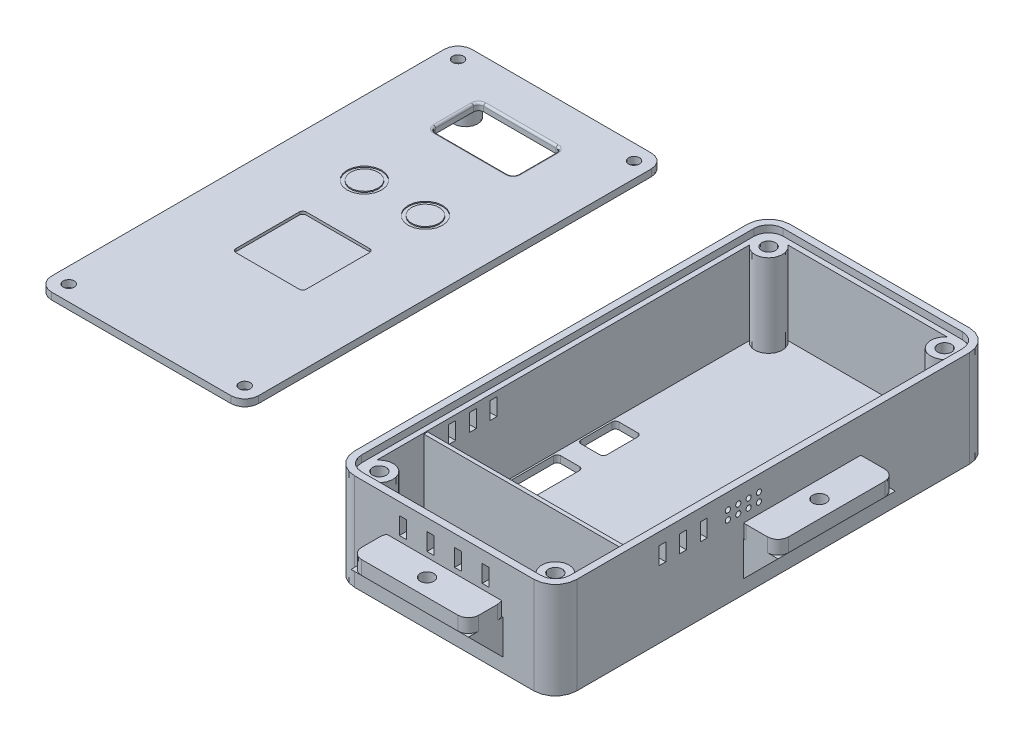
CARA_TEO (Autodesk Fusion 360 design; units mm, degrees)
part number: 2026-09-04-16-03-50-091
Autodesk Fusion 360 part; units mm, degrees
sketch "Boceto21" plane through (0, 0, 0) normal (0, 0, 1) x (1, 0, 0)
  line L0 (4, -16.8) -> (56, -16.8)
  line L1 (60, -12.8) -> (60, 101)
  line L2 (56, 105) -> (4, 105)
  line L3 (0, 101) -> (0, -12.8)
  arc A0 (56, -16.8) -> (60, -12.8) centre (56, -12.8) ccw
  arc A1 (60, 101) -> (56, 105) centre (56, 101) ccw
  arc A2 (4, 105) -> (0, 101) centre (4, 101) ccw
  arc A3 (0, -12.8) -> (4, -16.8) centre (4, -12.8) ccw
  constraint coincident L1.start A0.end
  constraint coincident L3.end A3.start
extrude "Extruir20" add sketch "Boceto21" along normal blind 2 makes body 1
sketch "Boceto22" plane through (0, 0, 0) normal (0, 0, 1) x (1, 0, 0)
  circle A0 centre (48.4706, 8.7122) radius 3.5
  circle A1 centre (11.3516, 8.7122) radius 3.5
  circle A2 centre (48.5136, 96.0852) radius 3.5
  circle A3 centre (11.0776, 96.1372) radius 3.5
extrude "Extruir21" add sketch "Boceto22" against normal blind 7 bodies 1
sketch "Boceto23" plane through (0, 0, 0) normal (0, 0, 1) x (1, 0, 0)
  circle A0 centre (48.4706, 8.7122) radius 1.25
  circle A1 centre (11.3516, 8.7122) radius 1.25
  circle A2 centre (48.5136, 96.0852) radius 1.25
  circle A3 centre (11.0776, 96.1372) radius 1.25
extrude "Extruir22" cut sketch "Boceto23" against normal blind 7 bodies 1
sketch "Boceto24" plane through (0, 0, 0) normal (0, 0, 1) x (1, 0, 0)
  circle A0 centre (4.5, -12.3) radius 1.6
  circle A1 centre (55.5, -12.3) radius 1.6
  circle A2 centre (4.5, 100.5) radius 1.6
  circle A3 centre (55.5, 100.5) radius 1.6
extrude "Extruir23" cut sketch "Boceto24" along normal blind 2 bodies 1
sketch "Boceto25" plane through (0, 0, 0) normal (0, 0, 1) x (1, 0, 0)
  line L0 (17.9336, 79.0164) -> (41.9336, 79.0164)
  line L1 (41.9336, 79.0164) -> (41.9336, 93.0164)
  line L2 (41.9336, 93.0164) -> (17.9336, 93.0164)
  line L3 (17.9336, 93.0164) -> (17.9336, 79.0164)
extrude "Extruir24" cut sketch "Boceto25" along normal blind 2 bodies 1
sketch "Boceto26" plane through (0, 0, 0) normal (0, 0, 1) x (1, 0, 0)
  line L0 (14.7446, 48.1164) -> (27.7446, 48.1164)
  line L1 (27.7446, 48.1164) -> (27.7446, 65.1164)
  line L2 (27.7446, 65.1164) -> (14.7446, 65.1164)
  line L3 (14.7446, 65.1164) -> (14.7446, 48.1164)
  line L4 (32.4246, 48.1164) -> (45.4246, 48.1164)
  line L5 (45.4246, 48.1164) -> (45.4246, 65.1164)
  line L6 (45.4246, 65.1164) -> (32.4246, 65.1164)
  line L7 (32.4246, 65.1164) -> (32.4246, 48.1164)
extrude "Extruir25" cut sketch "Boceto26" along normal blind 1.1 bodies 1
sketch "Boceto27" plane through (0, 0, 0) normal (0, 0, 1) x (1, 0, 0)
  line L0 (8.4354, 5.9164) -> (114.4697, 5.9164)
  line L1 (114.4697, 5.9164) -> (114.4697, 99.0836)
  line L2 (114.4697, 99.0836) -> (8.4354, 99.0836)
  line L3 (8.4354, 99.0836) -> (8.4354, 5.9164)
ref_plane "PlanoDeObra2" through (0, 0, 2) normal (0, 0, 1) x (1, 0, 0)
sketch "Boceto28" plane through (0, 0, 2) normal (0, 0, 1) x (1, 0, 0)
  line L0 (20.8, 19.8) -> (39.2, 19.8)
  line L1 (40.2, 20.8) -> (40.2, 39.2)
  line L2 (39.2, 40.2) -> (20.8, 40.2)
  line L3 (19.8, 39.2) -> (19.8, 20.8)
  arc A0 (39.2, 19.8) -> (40.2, 20.8) centre (39.2, 20.8) ccw
  arc A1 (40.2, 39.2) -> (39.2, 40.2) centre (39.2, 39.2) ccw
  arc A2 (20.8, 40.2) -> (19.8, 39.2) centre (20.8, 39.2) ccw
  arc A3 (19.8, 20.8) -> (20.8, 19.8) centre (20.8, 20.8) ccw
extrude "Extruir26" cut sketch "Boceto28" against normal blind 0.8 bodies 1
sketch "Boceto29" plane through (0, 0, 2) normal (0, 0, 1) x (1, 0, 0)
  circle A0 centre (21.2446, 56.6164) radius 5
  circle A1 centre (21.2446, 56.6164) radius 4
  line L0 (19.7446, 56.6164) -> (22.7446, 56.6164)
  line L1 (21.2446, 55.1164) -> (21.2446, 58.1164)
  circle A2 centre (38.9246, 56.6164) radius 5
  circle A3 centre (38.9246, 56.6164) radius 4
  line L2 (37.4246, 56.6164) -> (40.4246, 56.6164)
  line L3 (38.9246, 55.1164) -> (38.9246, 58.1164)
sketch "Boceto30" plane through (0, 0, 2) normal (0, 0, 1) x (1, 0, 0)
  circle A0 centre (21.2446, 56.6164) radius 5
  circle A1 centre (21.2446, 56.6164) radius 4
  circle A2 centre (38.9246, 56.6164) radius 5
  circle A3 centre (38.9246, 56.6164) radius 4
extrude "Extruir27" cut sketch "Boceto30" against normal blind 0.3 bodies 1
sketch "Boceto31" plane through (0, 0, 0) normal (0, 0, 1) x (1, 0, 0)
  line L0 (94, -19) -> (146, -19)
  line L1 (152.2, -12.8) -> (152.2, 101)
  line L2 (146, 107.2) -> (94, 107.2)
  line L3 (87.8, 101) -> (87.8, -12.8)
  arc A0 (146, -19) -> (152.2, -12.8) centre (146, -12.8) ccw
  arc A1 (152.2, 101) -> (146, 107.2) centre (146, 101) ccw
  arc A2 (94, 107.2) -> (87.8, 101) centre (94, 101) ccw
  arc A3 (87.8, -12.8) -> (94, -19) centre (94, -12.8) ccw
  constraint tangent L0 A0
  constraint tangent L1 A0
  constraint tangent L1 A1
  constraint tangent L2 A1
  constraint tangent L2 A2
  constraint tangent L3 A2
  constraint tangent L3 A3
  constraint tangent L0 A3
extrude "C_Cuerpo_macizo" add sketch "Boceto31" along normal blind 2 and the other way blind 26 separate body makes body 2
sketch "Boceto32" plane through (0, 0, 0) normal (0, 0, 1) x (1, 0, 0)
  line L0 (94, -17) -> (146, -17)
  line L1 (150.2, -12.8) -> (150.2, 101)
  line L2 (146, 105.2) -> (94, 105.2)
  line L3 (89.8, 101) -> (89.8, -12.8)
  arc A0 (146, -17) -> (150.2, -12.8) centre (146, -12.8) ccw
  arc A1 (150.2, 101) -> (146, 105.2) centre (146, 101) ccw
  arc A2 (94, 105.2) -> (89.8, 101) centre (94, 101) ccw
  arc A3 (89.8, -12.8) -> (94, -17) centre (94, -12.8) ccw
  constraint tangent L0 A0
  constraint tangent L1 A0
  constraint tangent L1 A1
  constraint tangent L2 A1
  constraint tangent L2 A2
  constraint tangent L3 A2
  constraint tangent L3 A3
  constraint tangent L0 A3
extrude "C_Rebaje_cara" cut sketch "Boceto32" along normal blind 2 bodies 2
sketch "Boceto33" plane through (0, 0, 0) normal (0, 0, 1) x (1, 0, 0)
  line L0 (94, -17) -> (146, -17)
  line L1 (148.7, -14.3) -> (148.7, 101)
  line L2 (146, 103.7) -> (94, 103.7)
  line L3 (91.3, 101) -> (91.3, -14.3)
  arc A0 (146, -17) -> (148.7, -14.3) centre (146, -14.3) ccw
  arc A1 (148.7, 101) -> (146, 103.7) centre (146, 101) ccw
  arc A2 (94, 103.7) -> (91.3, 101) centre (94, 101) ccw
  arc A3 (91.3, -14.3) -> (94, -17) centre (94, -14.3) ccw
  constraint tangent L0 A0
  constraint tangent L1 A0
  constraint tangent L1 A1
  constraint tangent L2 A1
  constraint tangent L2 A2
  constraint tangent L3 A2
  constraint tangent L3 A3
  constraint tangent L0 A3
extrude "C_Cavidad" cut sketch "Boceto33" against normal blind 24 bodies 2
sketch "Boceto34" plane through (0, 0, 0) normal (0, 0, 1) x (1, 0, 0)
  circle A0 centre (94.5, -12.3) radius 4
  circle A1 centre (145.5, -12.3) radius 4
  circle A2 centre (94.5, 100.5) radius 4
  circle A3 centre (145.5, 100.5) radius 4
extrude "C_Torres_esquina" add sketch "Boceto34" against normal blind 24 bodies 2
sketch "Boceto35" plane through (0, 0, 0) normal (0, 0, 1) x (1, 0, 0)
  circle A0 centre (94.5, -12.3) radius 2
  circle A1 centre (145.5, -12.3) radius 2
  circle A2 centre (94.5, 100.5) radius 2
  circle A3 centre (145.5, 100.5) radius 2
extrude "C_Pilotos_M3" cut sketch "Boceto35" against normal blind 10 bodies 2
move_body "C_Montaje_en_cara" bodies 2 to x (1, 0, 0) y (0, 1, 0) z (0, 0, 1) at (-90, 0, 0)
sketch "Boceto36" plane through (0, 0, 0) normal (1, 0, 0) x (0, 0, -1)
  line L0 (19.5, 15.9) -> (7.5, 15.9)
  line L1 (7.5, 15.9) -> (7.5, 41.9)
  line L2 (7.5, 41.9) -> (19.5, 41.9)
  line L3 (19.5, 41.9) -> (19.5, 15.9)
extrude "C_Hueco_borneras" [suppressed]
sketch "Boceto37" plane through (0, 0, 0) normal (1, 0, 0) x (0, 0, -1)
  line L0 (19.5, 43) -> (7.5, 43)
  line L1 (7.5, 43) -> (7.5, 59)
  line L2 (7.5, 59) -> (19.5, 59)
  line L3 (19.5, 59) -> (19.5, 43)
extrude "C_Hueco_USBC" [suppressed]
sketch "Boceto38" plane through (0, 0, 0) normal (1, 0, 0) x (0, 0, -1)
  line L0 (19.5, 16.55) -> (7.5, 16.55)
  line L1 (7.5, 16.55) -> (7.5, 26.85)
  line L2 (7.5, 26.85) -> (19.5, 26.85)
  line L3 (19.5, 26.85) -> (19.5, 16.55)
extrude "C_Hueco_alimentacion" [suppressed]
move_body "C_Separar_piezas" bodies 2 to x (1, 0, 0) y (0, 1, 0) z (0, 0, 1) at (90, 0, 0)
sketch "Boceto39" plane through (0, 0, 0) normal (1, 0, 0) x (0, 0, -1)
  line L0 (19.5, 47.8) -> (7.5, 47.8)
  line L1 (7.5, 47.8) -> (7.5, 58.8)
  line L2 (7.5, 58.8) -> (19.5, 58.8)
  line L3 (19.5, 58.8) -> (19.5, 47.8)
extrude "C_Hueco_sensor" [suppressed]
sketch "Boceto40" plane through (0, 0, 0) normal (0, 0, 1) x (1, 0, 0)
  line L0 (106, -29) -> (134, -29)
  line L1 (137, -26) -> (137, -20.5)
  line L2 (134, -17.5) -> (106, -17.5)
  line L3 (103, -20.5) -> (103, -26)
  arc A0 (134, -29) -> (137, -26) centre (134, -26) ccw
  arc A1 (137, -20.5) -> (134, -17.5) centre (134, -20.5) ccw
  arc A2 (106, -17.5) -> (103, -20.5) centre (106, -20.5) ccw
  arc A3 (103, -26) -> (106, -29) centre (106, -26) ccw
  line L4 (106, 105) -> (134, 105)
  line L5 (137, 108) -> (137, 114.2)
  line L6 (134, 117.2) -> (106, 117.2)
  line L7 (103, 114.2) -> (103, 108)
  arc A4 (134, 105) -> (137, 108) centre (134, 108) ccw
  arc A5 (137, 114.2) -> (134, 117.2) centre (134, 114.2) ccw
  arc A6 (106, 117.2) -> (103, 114.2) centre (106, 114.2) ccw
  arc A7 (103, 108) -> (106, 105) centre (106, 108) ccw
  constraint tangent L0 A0
  constraint tangent L1 A0
  constraint tangent L1 A1
  constraint tangent L2 A1
  constraint tangent L2 A2
  constraint tangent L3 A2
  constraint tangent L3 A3
  constraint tangent L0 A3
  constraint tangent L4 A4
  constraint tangent L5 A4
  constraint tangent L5 A5
  constraint tangent L6 A5
  constraint tangent L6 A6
  constraint tangent L7 A6
  constraint tangent L7 A7
  constraint tangent L4 A7
extrude "C_Orejas_correa" add sketch "Boceto40" along normal blind 4 from surface at -12 bodies 2
sketch "Boceto41" plane through (0, 0, 0) normal (0, 0, 1) x (1, 0, 0)
  line L0 (108.5, -9.2) -> (131.5, -9.2)
  line L1 (133, -7.7) -> (133, -6.7)
  line L2 (131.5, -5.2) -> (108.5, -5.2)
  line L3 (107, -6.7) -> (107, -7.7)
  arc A0 (131.5, -9.2) -> (133, -7.7) centre (131.5, -7.7) ccw
  arc A1 (133, -6.7) -> (131.5, -5.2) centre (131.5, -6.7) ccw
  arc A2 (108.5, -5.2) -> (107, -6.7) centre (108.5, -6.7) ccw
  arc A3 (107, -7.7) -> (108.5, -9.2) centre (108.5, -7.7) ccw
  line L4 (108.5, 110.2) -> (131.5, 110.2)
  line L5 (133, 111.7) -> (133, 112.7)
  line L6 (131.5, 114.2) -> (108.5, 114.2)
  line L7 (107, 112.7) -> (107, 111.7)
  arc A4 (131.5, 110.2) -> (133, 111.7) centre (131.5, 111.7) ccw
  arc A5 (133, 112.7) -> (131.5, 114.2) centre (131.5, 112.7) ccw
  arc A6 (108.5, 114.2) -> (107, 112.7) centre (108.5, 112.7) ccw
  arc A7 (107, 111.7) -> (108.5, 110.2) centre (108.5, 111.7) ccw
  constraint tangent L0 A0
  constraint tangent L1 A0
  constraint tangent L1 A1
  constraint tangent L2 A1
  constraint tangent L2 A2
  constraint tangent L3 A2
  constraint tangent L3 A3
  constraint tangent L0 A3
  constraint tangent L4 A4
  constraint tangent L5 A4
  constraint tangent L5 A5
  constraint tangent L6 A5
  constraint tangent L6 A6
  constraint tangent L7 A6
  constraint tangent L7 A7
  constraint tangent L4 A7
extrude "C_Ranuras_correa" [suppressed]
delete_face "SuprimirCaras1" [suppressed]
sketch "Boceto42" plane through (0, 0, 0) normal (0, 0, 1) x (1, 0, 0)
  line L0 (80.8, 35.5) -> (87, 35.5)
  line L1 (90, 38.5) -> (90, 66.5)
  line L2 (87, 69.5) -> (80.8, 69.5)
  line L3 (77.8, 66.5) -> (77.8, 38.5)
  arc A0 (87, 35.5) -> (90, 38.5) centre (87, 38.5) ccw
  arc A1 (90, 66.5) -> (87, 69.5) centre (87, 66.5) ccw
  arc A2 (80.8, 69.5) -> (77.8, 66.5) centre (80.8, 66.5) ccw
  arc A3 (77.8, 38.5) -> (80.8, 35.5) centre (80.8, 38.5) ccw
  line L4 (153, 35.5) -> (159.2, 35.5)
  line L5 (162.2, 38.5) -> (162.2, 66.5)
  line L6 (159.2, 69.5) -> (153, 69.5)
  line L7 (150, 66.5) -> (150, 38.5)
  arc A4 (159.2, 35.5) -> (162.2, 38.5) centre (159.2, 38.5) ccw
  arc A5 (162.2, 66.5) -> (159.2, 69.5) centre (159.2, 66.5) ccw
  arc A6 (153, 69.5) -> (150, 66.5) centre (153, 66.5) ccw
  arc A7 (150, 38.5) -> (153, 35.5) centre (153, 38.5) ccw
  constraint tangent L0 A0
  constraint tangent L1 A0
  constraint tangent L1 A1
  constraint tangent L2 A1
  constraint tangent L2 A2
  constraint tangent L3 A2
  constraint tangent L3 A3
  constraint tangent L0 A3
  constraint tangent L4 A4
  constraint tangent L5 A4
  constraint tangent L5 A5
  constraint tangent L6 A5
  constraint tangent L6 A6
  constraint tangent L7 A6
  constraint tangent L7 A7
  constraint tangent L4 A7
extrude "C_Orejas_laterales" add sketch "Boceto42" along normal blind 4 from surface at -12 bodies 2
sketch "Boceto43" plane through (0, 0, 0) normal (0, 0, 1) x (1, 0, 0)
  line L0 (82.3, 39.5) -> (83.3, 39.5)
  line L1 (84.8, 41) -> (84.8, 64)
  line L2 (83.3, 65.5) -> (82.3, 65.5)
  line L3 (80.8, 64) -> (80.8, 41)
  arc A0 (83.3, 39.5) -> (84.8, 41) centre (83.3, 41) ccw
  arc A1 (84.8, 64) -> (83.3, 65.5) centre (83.3, 64) ccw
  arc A2 (82.3, 65.5) -> (80.8, 64) centre (82.3, 64) ccw
  arc A3 (80.8, 41) -> (82.3, 39.5) centre (82.3, 41) ccw
  line L4 (156.7, 39.5) -> (157.7, 39.5)
  line L5 (159.2, 41) -> (159.2, 64)
  line L6 (157.7, 65.5) -> (156.7, 65.5)
  line L7 (155.2, 64) -> (155.2, 41)
  arc A4 (157.7, 39.5) -> (159.2, 41) centre (157.7, 41) ccw
  arc A5 (159.2, 64) -> (157.7, 65.5) centre (157.7, 64) ccw
  arc A6 (156.7, 65.5) -> (155.2, 64) centre (156.7, 64) ccw
  arc A7 (155.2, 41) -> (156.7, 39.5) centre (156.7, 41) ccw
  constraint tangent L0 A0
  constraint tangent L1 A0
  constraint tangent L1 A1
  constraint tangent L2 A1
  constraint tangent L2 A2
  constraint tangent L3 A2
  constraint tangent L3 A3
  constraint tangent L0 A3
  constraint tangent L4 A4
  constraint tangent L5 A4
  constraint tangent L5 A5
  constraint tangent L6 A5
  constraint tangent L6 A6
  constraint tangent L7 A6
  constraint tangent L7 A7
  constraint tangent L4 A7
extrude "C_Ranuras_laterales" [suppressed]
sketch "Boceto44" plane through (0, 0, 0) normal (0, 0, 1) x (1, 0, 0)
  line L0 (94, -0.2) -> (146, -0.2)
  line L1 (150.2, 4) -> (150.2, 101)
  line L2 (146, 105.2) -> (94, 105.2)
  line L3 (89.8, 101) -> (89.8, 4)
  arc A0 (146, -0.2) -> (150.2, 4) centre (146, 4) ccw
  arc A1 (150.2, 101) -> (146, 105.2) centre (146, 101) ccw
  arc A2 (94, 105.2) -> (89.8, 101) centre (94, 101) ccw
  arc A3 (89.8, 4) -> (94, -0.2) centre (94, 4) ccw
  constraint tangent L0 A0
  constraint tangent L1 A0
  constraint tangent L1 A1
  constraint tangent L2 A1
  constraint tangent L2 A2
  constraint tangent L3 A2
  constraint tangent L3 A3
  constraint tangent L0 A3
extrude "C_Rebaje_limpieza" [suppressed]
move_body "C_Montaje_final" bodies 2 to x (1, 0, 0) y (0, 1, 0) z (0, 0, 1) at (-90, 0, 0)
move_body "C_Separar_vista" bodies 2 to x (1, 0, 0) y (0, 1, 0) z (0, 0, 1) at (90, 0, 0)
sketch "Boceto45" plane through (0, 0, 0) normal (0, 0, 1) x (1, 0, 0)
  line L0 (92.8, 15.9) -> (98.3, 15.9)
  line L1 (99.3, 16.9) -> (99.3, 40.9)
  line L2 (98.3, 41.9) -> (92.8, 41.9)
  line L3 (91.8, 40.9) -> (91.8, 16.9)
  arc A0 (98.3, 15.9) -> (99.3, 16.9) centre (98.3, 16.9) ccw
  arc A1 (99.3, 40.9) -> (98.3, 41.9) centre (98.3, 40.9) ccw
  arc A2 (92.8, 41.9) -> (91.8, 40.9) centre (92.8, 40.9) ccw
  arc A3 (91.8, 16.9) -> (92.8, 15.9) centre (92.8, 16.9) ccw
  line L4 (92.8, 47.8) -> (98.3, 47.8)
  line L5 (99.3, 48.8) -> (99.3, 57.8)
  line L6 (98.3, 58.8) -> (92.8, 58.8)
  line L7 (91.8, 57.8) -> (91.8, 48.8)
  arc A4 (98.3, 47.8) -> (99.3, 48.8) centre (98.3, 48.8) ccw
  arc A5 (99.3, 57.8) -> (98.3, 58.8) centre (98.3, 57.8) ccw
  arc A6 (92.8, 58.8) -> (91.8, 57.8) centre (92.8, 57.8) ccw
  arc A7 (91.8, 48.8) -> (92.8, 47.8) centre (92.8, 48.8) ccw
  line L8 (141.7, 15.9) -> (147.2, 15.9)
  line L9 (148.2, 16.9) -> (148.2, 40.9)
  line L10 (147.2, 41.9) -> (141.7, 41.9)
  line L11 (140.7, 40.9) -> (140.7, 16.9)
  arc A8 (147.2, 15.9) -> (148.2, 16.9) centre (147.2, 16.9) ccw
  arc A9 (148.2, 40.9) -> (147.2, 41.9) centre (147.2, 40.9) ccw
  arc A10 (141.7, 41.9) -> (140.7, 40.9) centre (141.7, 40.9) ccw
  arc A11 (140.7, 16.9) -> (141.7, 15.9) centre (141.7, 16.9) ccw
  line L12 (141.7, 47.8) -> (147.2, 47.8)
  line L13 (148.2, 48.8) -> (148.2, 57.8)
  line L14 (147.2, 58.8) -> (141.7, 58.8)
  line L15 (140.7, 57.8) -> (140.7, 48.8)
  arc A12 (147.2, 47.8) -> (148.2, 48.8) centre (147.2, 48.8) ccw
  arc A13 (148.2, 57.8) -> (147.2, 58.8) centre (147.2, 57.8) ccw
  arc A14 (141.7, 58.8) -> (140.7, 57.8) centre (141.7, 57.8) ccw
  arc A15 (140.7, 48.8) -> (141.7, 47.8) centre (141.7, 48.8) ccw
  constraint tangent L0 A0
  constraint tangent L1 A0
  constraint tangent L1 A1
  constraint tangent L2 A1
  constraint tangent L2 A2
  constraint tangent L3 A2
  constraint tangent L3 A3
  constraint tangent L0 A3
  constraint tangent L4 A4
  constraint tangent L5 A4
  constraint tangent L5 A5
  constraint tangent L6 A5
  constraint tangent L6 A6
  constraint tangent L7 A6
  constraint tangent L7 A7
  constraint tangent L4 A7
  constraint tangent L8 A8
  constraint tangent L9 A8
  constraint tangent L9 A9
  constraint tangent L10 A9
  constraint tangent L10 A10
  constraint tangent L11 A10
  constraint tangent L11 A11
  constraint tangent L8 A11
  constraint tangent L12 A12
  constraint tangent L13 A12
  constraint tangent L13 A13
  constraint tangent L14 A13
  constraint tangent L14 A14
  constraint tangent L15 A14
  constraint tangent L15 A15
  constraint tangent L12 A15
extrude "C_Salidas_fondo" cut sketch "Boceto45" along normal blind 4 from surface at -27 bodies 2
sketch "Boceto46" plane through (0, 0, 0) normal (0, 0, 1) x (1, 0, 0)
  circle A0 centre (120, -24) radius 2
  circle A1 centre (120, 112.2) radius 2
  circle A2 centre (82.8, 52.5) radius 2
  circle A3 centre (157.2, 52.5) radius 2
extrude "C_Huecos_tornillo_orejas" cut sketch "Boceto46" along normal blind 6 from surface at -13 bodies 2
fillet "Redondeo_esquinas_OLED" radius 1.5 4 edges at (41.9336, 93.0164, 1) (17.9336, 93.0164, 1) (41.9336, 79.0164, 1) (17.9336, 79.0164, 1) on bodies 1
fillet "Suavizado_borde_OLED" radius 0.6 64 edges at (18.3729, 79.4557, 2) (29.9336, 79.0164, 2) (41.4943, 79.4557, 2) (41.9336, 86.0164, 2) (41.4943, 92.5771, 2) (29.9336, 93.0164, 2) (18.3729, 92.5771, 2) (17.9336, 86.0164, 2) (17.9336, 86.0164, 2) (18.3729, 92.5771, 2) (29.9336, 93.0164, 2) (41.4943, 92.5771, 2) (41.9336, 86.0164, 2) (41.4943, 79.4557, 2) (29.9336, 79.0164, 2) (18.3729, 79.4557, 2) (41.4943, 79.4557, 2) (41.9336, 86.0164, 2) (41.4943, 92.5771, 2) (29.9336, 93.0164, 2) (18.3729, 92.5771, 2) (17.9336, 86.0164, 2) (18.3729, 79.4557, 2) (29.9336, 79.0164, 2) (29.9336, 79.0164, 2) (18.3729, 79.4557, 2) (17.9336, 86.0164, 2) (18.3729, 92.5771, 2) (29.9336, 93.0164, 2) (41.4943, 92.5771, 2) (41.9336, 86.0164, 2) (41.4943, 79.4557, 2) (18.3729, 92.5771, 2) (17.9336, 86.0164, 2) (18.3729, 79.4557, 2) (29.9336, 79.0164, 2) (41.4943, 79.4557, 2) (41.9336, 86.0164, 2) (41.4943, 92.5771, 2) (29.9336, 93.0164, 2) (29.9336, 93.0164, 2) (41.4943, 92.5771, 2) (41.9336, 86.0164, 2) (41.4943, 79.4557, 2) (29.9336, 79.0164, 2) (18.3729, 79.4557, 2) (17.9336, 86.0164, 2) (18.3729, 92.5771, 2) (41.4943, 92.5771, 2) (29.9336, 93.0164, 2) (18.3729, 92.5771, 2) (17.9336, 86.0164, 2) (18.3729, 79.4557, 2) (29.9336, 79.0164, 2) (41.4943, 79.4557, 2) (41.9336, 86.0164, 2) (41.9336, 86.0164, 2) (41.4943, 79.4557, 2) (29.9336, 79.0164, 2) (18.3729, 79.4557, 2) (17.9336, 86.0164, 2) (18.3729, 92.5771, 2) (29.9336, 93.0164, 2) (41.4943, 92.5771, 2) on bodies 1
sketch "Boceto47" plane through (0, 0, 0) normal (0, 0, 1) x (1, 0, 0)
  line L0 (90.8, -14.3) -> (94.5, -14.3)
  line L1 (94.5, -14.3) -> (94.5, -10.3)
  line L2 (94.5, -10.3) -> (90.8, -10.3)
  line L3 (90.8, -10.3) -> (90.8, -14.3)
  line L4 (145.5, -14.3) -> (149.2, -14.3)
  line L5 (149.2, -14.3) -> (149.2, -10.3)
  line L6 (149.2, -10.3) -> (145.5, -10.3)
  line L7 (145.5, -10.3) -> (145.5, -14.3)
  line L8 (90.8, 98.5) -> (94.5, 98.5)
  line L9 (94.5, 98.5) -> (94.5, 102.5)
  line L10 (94.5, 102.5) -> (90.8, 102.5)
  line L11 (90.8, 102.5) -> (90.8, 98.5)
  line L12 (145.5, 98.5) -> (149.2, 98.5)
  line L13 (149.2, 98.5) -> (149.2, 102.5)
  line L14 (149.2, 102.5) -> (145.5, 102.5)
  line L15 (145.5, 102.5) -> (145.5, 98.5)
  line L16 (92.5, 100.5) -> (96.5, 100.5)
  line L17 (96.5, 100.5) -> (96.5, 104.2)
  line L18 (96.5, 104.2) -> (92.5, 104.2)
  line L19 (92.5, 104.2) -> (92.5, 100.5)
  line L20 (143.5, 100.5) -> (147.5, 100.5)
  line L21 (147.5, 100.5) -> (147.5, 104.2)
  line L22 (147.5, 104.2) -> (143.5, 104.2)
  line L23 (143.5, 104.2) -> (143.5, 100.5)
extrude "C_Union_torres_pared" add sketch "Boceto47" against normal blind 24 bodies 2
sketch "Boceto48" plane through (0, 0, 0) normal (0, 0, 1) x (1, 0, 0)
  circle A0 centre (94.5, -12.3) radius 2
  circle A1 centre (145.5, -12.3) radius 2
  circle A2 centre (94.5, 100.5) radius 2
  circle A3 centre (145.5, 100.5) radius 2
extrude "C_Pilotos_repaso" cut sketch "Boceto48" against normal blind 10 bodies 2
sketch "Boceto49" plane through (0, 0, 0) normal (0, 0, 1) x (1, 0, 0)
  line L0 (92.5, -17.5) -> (96.5, -17.5)
  line L1 (96.5, -17.5) -> (96.5, -12.3)
  line L2 (96.5, -12.3) -> (92.5, -12.3)
  line L3 (92.5, -12.3) -> (92.5, -17.5)
  line L4 (143.5, -17.5) -> (147.5, -17.5)
  line L5 (147.5, -17.5) -> (147.5, -12.3)
  line L6 (147.5, -12.3) -> (143.5, -12.3)
  line L7 (143.5, -12.3) -> (143.5, -17.5)
extrude "C_Union_torres_extremo" add sketch "Boceto49" against normal blind 24 bodies 2
sketch "Boceto50" plane through (0, 0, 0) normal (0, 0, 1) x (1, 0, 0)
  circle A0 centre (94.5, -12.3) radius 2
  circle A1 centre (145.5, -12.3) radius 2
extrude "C_Pilotos_repaso_extremo" cut sketch "Boceto50" against normal blind 10 bodies 2
sketch "Boceto51" plane through (0, 0, 0) normal (1, 0, 0) x (0, 0, -1)
  circle A0 centre (2.5, 31) radius 0.75
  circle A1 centre (5, 31) radius 0.75
  circle A2 centre (2.5, 34) radius 0.75
  circle A3 centre (5, 34) radius 0.75
  circle A4 centre (2.5, 37) radius 0.75
  circle A5 centre (5, 37) radius 0.75
  circle A6 centre (2.5, 40) radius 0.75
  circle A7 centre (5, 40) radius 0.75
extrude "C_Agujeros_buzzer" cut sketch "Boceto51" along normal blind 10 from surface at 146 bodies 2
sketch "Boceto52" plane through (0, 0, 0) normal (1, 0, 0) x (0, 0, -1)
  line L0 (6.5, 11) -> (1.5, 11)
  line L1 (1.5, 11) -> (1.5, 13)
  line L2 (1.5, 13) -> (6.5, 13)
  line L3 (6.5, 13) -> (6.5, 11)
  line L4 (6.5, 17) -> (1.5, 17)
  line L5 (1.5, 17) -> (1.5, 19)
  line L6 (1.5, 19) -> (6.5, 19)
  line L7 (6.5, 19) -> (6.5, 17)
  line L8 (6.5, 23) -> (1.5, 23)
  line L9 (1.5, 23) -> (1.5, 25)
  line L10 (1.5, 25) -> (6.5, 25)
  line L11 (6.5, 25) -> (6.5, 23)
extrude "C_Ventilacion_lat_Xmenos" cut sketch "Boceto52" along normal blind 10 from surface at 84 bodies 2
sketch "Boceto53" plane through (0, 0, 0) normal (1, 0, 0) x (0, 0, -1)
  line L0 (6.5, 11) -> (1.5, 11)
  line L1 (1.5, 11) -> (1.5, 13)
  line L2 (1.5, 13) -> (6.5, 13)
  line L3 (6.5, 13) -> (6.5, 11)
  line L4 (6.5, 17) -> (1.5, 17)
  line L5 (1.5, 17) -> (1.5, 19)
  line L6 (1.5, 19) -> (6.5, 19)
  line L7 (6.5, 19) -> (6.5, 17)
  line L8 (6.5, 23) -> (1.5, 23)
  line L9 (1.5, 23) -> (1.5, 25)
  line L10 (1.5, 25) -> (6.5, 25)
  line L11 (6.5, 25) -> (6.5, 23)
extrude "C_Ventilacion_lat_Xmas" cut sketch "Boceto53" along normal blind 10 from surface at 146 bodies 2
ref_plane "PlanoDeObra3" through (0, -18, 0) normal (0, 1, 0) x (0, 0, 1)
sketch "Boceto54" plane through (0, -18, 0) normal (0, 1, 0) x (1, 0, 0)
  line L0 (107, 6.5) -> (109, 6.5)
  line L1 (109, 6.5) -> (109, 1.5)
  line L2 (109, 1.5) -> (107, 1.5)
  line L3 (107, 1.5) -> (107, 6.5)
  line L4 (115, 6.5) -> (117, 6.5)
  line L5 (117, 6.5) -> (117, 1.5)
  line L6 (117, 1.5) -> (115, 1.5)
  line L7 (115, 1.5) -> (115, 6.5)
  line L8 (123, 6.5) -> (125, 6.5)
  line L9 (125, 6.5) -> (125, 1.5)
  line L10 (125, 1.5) -> (123, 1.5)
  line L11 (123, 1.5) -> (123, 6.5)
  line L12 (131, 6.5) -> (133, 6.5)
  line L13 (133, 6.5) -> (133, 1.5)
  line L14 (133, 1.5) -> (131, 1.5)
  line L15 (131, 1.5) -> (131, 6.5)
extrude "C_Ventilacion_convertidor" cut sketch "Boceto54" along normal mid plane 6 bodies 2
sketch "Boceto55" plane through (0, 0, 0) normal (1, 0, 0) x (0, 0, -1)
  line L0 (12, -18.5) -> (12, -29)
  line L1 (12, -29) -> (22.5, -18.5)
  line L2 (22.5, -18.5) -> (12, -18.5)
extrude "C_Nervio_nervio_extremo_conv_13" add sketch "Boceto55" along normal blind 3 from surface at 103 bodies 2
extrude "C_Nervio_nervio_extremo_conv_44" add sketch "Boceto55" along normal blind 3 from surface at 134 bodies 2
sketch "Boceto56" plane through (0, 0, 0) normal (1, 0, 0) x (0, 0, -1)
  line L0 (12, 106.7) -> (12, 117.2)
  line L1 (12, 117.2) -> (22.5, 106.7)
  line L2 (22.5, 106.7) -> (12, 106.7)
extrude "C_Nervio_nervio_extremo_OLED_13" add sketch "Boceto56" along normal blind 3 from surface at 103 bodies 2
extrude "C_Nervio_nervio_extremo_OLED_44" add sketch "Boceto56" along normal blind 3 from surface at 134 bodies 2
ref_plane "PlanoDeObra4" through (0, 37, 0) normal (0, 1, 0) x (0, 0, 1)
sketch "Boceto57" plane through (0, 37, 0) normal (0, 1, 0) x (1, 0, 0)
  line L0 (88.3, 12) -> (77.8, 12)
  line L1 (77.8, 12) -> (88.3, 22.5)
  line L2 (88.3, 22.5) -> (88.3, 12)
  line L3 (151.7, 12) -> (162.2, 12)
  line L4 (162.2, 12) -> (151.7, 22.5)
  line L5 (151.7, 22.5) -> (151.7, 12)
extrude "C_Nervios_laterales_a" add sketch "Boceto57" along normal mid plane 3 bodies 2
ref_plane "PlanoDeObra5" through (0, 68, 0) normal (0, 1, 0) x (0, 0, 1)
sketch "Boceto58" plane through (0, 68, 0) normal (0, 1, 0) x (1, 0, 0)
  line L0 (88.3, 12) -> (77.8, 12)
  line L1 (77.8, 12) -> (88.3, 22.5)
  line L2 (88.3, 22.5) -> (88.3, 12)
  line L3 (151.7, 12) -> (162.2, 12)
  line L4 (162.2, 12) -> (151.7, 22.5)
  line L5 (151.7, 22.5) -> (151.7, 12)
extrude "C_Nervios_laterales_b" add sketch "Boceto58" along normal mid plane 3 bodies 2
sketch "Boceto59" plane through (0, 0, 0) normal (0, 0, 1) x (1, 0, 0)
  line L0 (139.7, 20.5) -> (149.2, 20.5)
  line L1 (149.2, 20.5) -> (149.2, 23.5)
  line L2 (149.2, 23.5) -> (139.7, 23.5)
  line L3 (139.7, 23.5) -> (139.7, 20.5)
  line L4 (139.7, 34.5) -> (149.2, 34.5)
  line L5 (149.2, 34.5) -> (149.2, 37.5)
  line L6 (149.2, 37.5) -> (139.7, 37.5)
  line L7 (139.7, 37.5) -> (139.7, 34.5)
extrude "C_Anclajes_brida_120V" add sketch "Boceto59" along normal blind 2.5 from surface at -24 bodies 2
sketch "Boceto60" plane through (0, 0, 0) normal (0, 0, 1) x (1, 0, 0)
  line L0 (91, 3.8) -> (149, 3.8)
  line L1 (149, 3.8) -> (149, 4.9)
  line L2 (149, 4.9) -> (91, 4.9)
  line L3 (91, 4.9) -> (91, 3.8)
extrude "C_Barrera_convertidor" add sketch "Boceto60" along normal blind 24.2 from surface at -24.5 bodies 2
equation "fr_w = 60 mm" comment "FIRME  ancho del frontal"
equation "fr_h = 105 mm" comment "PENDIENTE  alto del frontal"
equation "fr_t = 2.0 mm" comment "espesor del frontal (subido de 1.5 para poder grabar)"
equation "fr_r = 4 mm" comment "PENDIENTE  radio de esquinas"
equation "col_H = 7 mm" comment "PROVISIONAL  col_H = M30 - (fr_t - pared_touch) = M30 - 1.1"
equation "col_od = 7 mm" comment "diametro exterior columna"
equation "col_id = 2.5 mm" comment "pilotaje M3 autorroscante"
equation "pared_touch = 0.9 mm" comment "pared sobre el touch antes del grabado"
equation "tor_frontal = 3.2 mm" comment "PENDIENTE  hueco tornillo de esquina"
equation "qr_lado = 20 mm" comment "lado de la etiqueta QR"
equation "qr_holgura = 0.4 mm" comment "holgura total del alojamiento"
equation "qr_prof = 0.8 mm" comment "profundidad del rebaje del QR (subida de 0.4 para que se perciba)"
equation "qr_cy = 30 mm" comment "altura del centro del QR sobre el borde inferior"
equation "d54 = fr_t"
equation "d56 = -col_H"
equation "d58 = -col_H"
equation "d60 = fr_t"
equation "d62 = fr_t"
equation "d64 = fr_t - pared_touch"
equation "d66 = fr_t"
equation "d68 = -qr_prof"
equation "anillo_ext = 10 mm" comment "diametro exterior del anillo guia"
equation "anillo_int = 8 mm" comment "diametro interior del anillo guia"
equation "anillo_prof = 0.3 mm" comment "profundidad del grabado del anillo"
equation "d73 = -anillo_prof"
named bodies: "Frontal", "Cuerpo"
